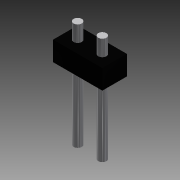
# Autodesk Inventor part: 2PinHeader
Saved by Autodesk Inventor 2014 (Build 180170000, 170)
## iProperties
Created: 2015-04-18
Part Number: 2PinHeader
Material: Generic
Document SubType Name: Modeling
Designer: Owner
Density: 1 g/cm^3
Appearance: Default
Author: Owner
Autodesk Inventor part; units mm, degrees
ref_plane "YZ Plane" through (0, 0, 0) normal (1, 0, 0) x (0, 1, 0)
ref_plane "XZ Plane" through (0, 0, 0) normal (0, 1, 0) x (-1, 0, 0)
sketch "Sketch1" plane through (0, 0, 0) normal (0, 1, 0) x (-1, 0, 0)
  circle A0 centre (0, 0) radius 0.4191
  circle A1 centre (2.54, 0) radius 0.4191
  circle A2 centre (-2.54, 0) radius 0.4191
  dimension "d0" = 0.8382
  dimension "d1" = 0.8382
  dimension "d2" = 0.8382
  dimension "d3" = 2.54
  dimension "d4" = 2.54
  constraints: 3 centre point, 1 coincident
  measures "d0" diameter of A2
  measures "d1" diameter of A0
  measures "d2" diameter of A1
  measures "d3" distance of A1.centre point (0, 0)
  measures "d4" distance of A2.centre point (0, 0)
extrude "Extrusion1" add sketch "Sketch1" along normal blind 11 contours A0 | A2
ref_plane "Work Plane1" through (2.54, 9.35, 0) normal (0, 1, 0) x (1, 0, 0)
sketch "Sketch2" plane through (2.54, 9.35, 0) normal (0, 1, 0) x (1, 0, 0)
  line L0 (-3.81, 1.27) -> (1.27, 1.27)
  line L1 (1.27, 1.27) -> (1.27, -1.27)
  line L2 (1.27, -1.27) -> (-3.81, -1.27)
  line L3 (-3.81, -1.27) -> (-3.81, 1.27)
  point P0 (-2.54, 0)
  dimension "d8" = 3.81
  dimension "d9" = 1.27
  dimension "d10" = 1.27
  dimension "d11" = 2.54
  constraints: 8 end point, 2 parallel, 1 horizontal, 1 perpendicular
  measures "d8" distance from line of L1 point (-2.54, 0)
  measures "d9" distance from line of L3 point (-2.54, 0)
  measures "d10" distance from line of point (-2.54, 0) L0
  measures "d11" distance of L0.end L1.end
extrude "Extrusion2" add sketch "Sketch2" against normal blind 2
body "Solid1"
